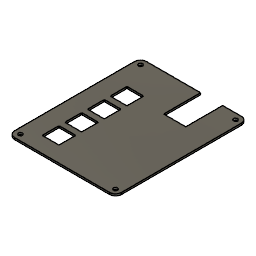
top hackpad (Autodesk Fusion 360 design; units mm, degrees)
part number: 2026-01-10-17-27-51-587
Autodesk Fusion 360 part; units mm, degrees
sketch "plate-2026-01-10T16_34_53.983Z" plane through (0, 0, 0) normal (0, 0, 1) x (1, 0, 0)
  line L0 (3.025, -21.575) -> (16.025, -21.575)
  line L1 (3.025, -35.575) -> (16.025, -35.575)
  line L2 (2.525, -22.075) -> (2.525, -35.075)
  line L3 (16.525, -22.075) -> (16.525, -35.075)
  arc A0 (3.025, -21.575) -> (2.525, -22.075) centre (3.025, -22.075) ccw
  arc A1 (16.525, -22.075) -> (16.025, -21.575) centre (16.025, -22.075) ccw
  arc A2 (2.525, -35.075) -> (3.025, -35.575) centre (3.025, -35.075) ccw
  arc A3 (16.025, -35.575) -> (16.525, -35.075) centre (16.025, -35.075) ccw
  line L4 (3.025, -40.625) -> (16.025, -40.625)
  line L5 (3.025, -54.625) -> (16.025, -54.625)
  line L6 (2.525, -41.125) -> (2.525, -54.125)
  line L7 (16.525, -41.125) -> (16.525, -54.125)
  arc A4 (3.025, -40.625) -> (2.525, -41.125) centre (3.025, -41.125) ccw
  arc A5 (16.525, -41.125) -> (16.025, -40.625) centre (16.025, -41.125) ccw
  arc A6 (2.525, -54.125) -> (3.025, -54.625) centre (3.025, -54.125) ccw
  arc A7 (16.025, -54.625) -> (16.525, -54.125) centre (16.025, -54.125) ccw
  line L8 (3.025, -59.675) -> (16.025, -59.675)
  line L9 (3.025, -73.675) -> (16.025, -73.675)
  line L10 (2.525, -60.175) -> (2.525, -73.175)
  line L11 (16.525, -60.175) -> (16.525, -73.175)
  arc A8 (3.025, -59.675) -> (2.525, -60.175) centre (3.025, -60.175) ccw
  arc A9 (16.525, -60.175) -> (16.025, -59.675) centre (16.025, -60.175) ccw
  arc A10 (2.525, -73.175) -> (3.025, -73.675) centre (3.025, -73.175) ccw
  arc A11 (16.025, -73.675) -> (16.525, -73.175) centre (16.025, -73.175) ccw
  line L12 (3.025, -78.725) -> (16.025, -78.725)
  line L13 (3.025, -92.725) -> (16.025, -92.725)
  line L14 (2.525, -79.225) -> (2.525, -92.225)
  line L15 (16.525, -79.225) -> (16.525, -92.225)
  arc A12 (3.025, -78.725) -> (2.525, -79.225) centre (3.025, -79.225) ccw
  arc A13 (16.525, -79.225) -> (16.025, -78.725) centre (16.025, -79.225) ccw
  arc A14 (2.525, -92.225) -> (3.025, -92.725) centre (3.025, -92.225) ccw
  arc A15 (16.025, -92.725) -> (16.525, -92.225) centre (16.025, -92.225) ccw
  line L16 (-12.565, 4.91) -> (77.435, 4.91)
  line L17 (77.435, 4.91) -> (77.435, -106.09)
  line L18 (77.435, -106.09) -> (-12.565, -106.09)
  line L19 (-12.565, -106.09) -> (-12.565, 4.91)
  line L20 (38.056, 4.91) -> (56.556, 4.91)
  line L21 (56.556, 4.91) -> (56.556, -26.09)
  line L22 (56.556, -26.09) -> (38.056, -26.09)
  line L23 (38.056, -26.09) -> (38.056, 4.91)
  circle A16 centre (-7.565, -101.09) radius 1.7
  circle A17 centre (72.435, -101.09) radius 1.7
  circle A18 centre (72.435, -0.09) radius 1.7
  circle A19 centre (-7.565, -0.09) radius 1.7
  dimension "d1" = 111
  dimension "d2" = 90
  dimension "d3" = 15.09
  dimension "d4" = 13.365
  dimension "d5" = 18.5
  dimension "d6" = 31
  dimension "d7" = 50.621
  dimension "d8" = 3.4
  dimension "d9" = 5
  dimension "d10" = 5
  dimension "d11" = 3.4
  dimension "d12" = 5
  dimension "d13" = 5
  dimension "d14" = 3.4
  dimension "d15" = 5
  dimension "d16" = 5
  dimension "d17" = 3.4
  dimension "d18" = 5
  dimension "d19" = 5
  constraint horizontal L16
  constraint vertical L17
  constraint horizontal L18
  constraint vertical L19
  constraint horizontal L20
  constraint vertical L21
  constraint horizontal L22
  constraint vertical L23
  constraint coincident L16 L20.start
  measures "d1" distance of L16.start L18.end
  measures "d2" distance of L16.start L16.end
  measures "d3" distance of L14 L19
  measures "d4" distance of L13 L18
  measures "d5" distance of L21.end L22.end
  measures "d6" distance of L20.end L21.end
  measures "d7" distance of L19 L23
  measures "d8" diameter of A16
  measures "d9" distance of L19 A16.centre
  measures "d10" distance of L18 A16.centre
  measures "d11" diameter of A17
  measures "d12" distance of L17 A17.centre
  measures "d13" distance of L18 A17.centre
  measures "d14" diameter of A18
  measures "d15" distance of L17 A18.centre
  measures "d16" distance of L16 A18.centre
  measures "d17" diameter of A19
  measures "d18" distance of L16 A19.centre
  measures "d19" distance of L19 A19.centre
sketch "Sketch2" plane through (0, 0, 0) normal (0, 0, 1) x (1, 0, 0)
sketch "Sketch3" plane through (0, 0, 0) normal (0, 0, 1) x (1, 0, 0)
extrude "Extrude1" add sketch "plate-2026-01-10T16_34_53.983Z" along normal blind 1.5 contours L16 L17 L18 L19 L21 L22 L23
fillet "Fillet1" radius 5 1 edges at (77.435, -106.09, 0.75)
fillet "Fillet2" radius 5 1 edges at (77.435, 4.91, 0.75)
fillet "Fillet3" radius 5 1 edges at (-12.565, 4.91, 0.75)
fillet "Fillet4" radius 5 1 edges at (-12.565, -106.09, 0.75)
